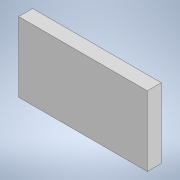
# Autodesk Inventor part: Ground3
Saved by Autodesk Inventor 2021 (Build 250183000, 183)
## iProperties
Created: 2022-07-02
Part Number: Ground3
Material: 一般
Document SubType Name: Modeling
Designer: tazak
Density: 1 g/cm^3
Appearance: 既定
Author: tazak
Autodesk Inventor part; units mm, degrees
ref_plane "YZ Plane" through (0, 0, 0) normal (1, 0, 0) x (0, 1, 0)
ref_plane "XZ Plane" through (0, 0, 0) normal (0, 1, 0) x (-1, 0, 0)
ref_plane "XY Plane" through (0, 0, 0) normal (0, 0, 1) x (1, 0, 0)
sketch "スケッチ1" plane through (0, 0, 0) normal (0, 0, 1) x (1, 0, 0)
  line L0 (4800, 2500) -> (14000, 2500)
  line L1 (14000, 2500) -> (14000, -2500)
  line L2 (14000, -2500) -> (4800, -2500)
  line L3 (4800, -2500) -> (4800, 2500)
  point P0 (0, 0)
  point P1 (4800, 0)
  dimension "d2" = 5000
  dimension "d5" = 4800
  dimension "d6" = 9200
  constraints: 8 end point, 2 parallel, 1 horizontal, 1 horizontal alignment, 1 midpoint, 1 perpendicular
  measures "d2" distance of L2.end L0.start
  measures "d5" distance from line of L3 point (0, 0)
  measures "d6" distance of L0.start L0.end
extrude "押し出し1" add sketch "スケッチ1" against normal blind 1000
